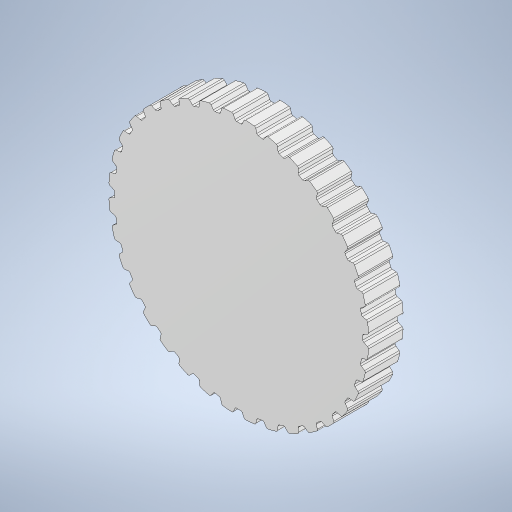
# Autodesk Inventor part: XL Pulley Generator
Saved by Autodesk Inventor 2023.4 (Build 274418000, 418)
## iProperties
RuleStatus: InUse
Created: 2022-06-22
Part Number: XL Pulley Generator
Material: UHMW, White
Document SubType Name: Modeling
Designer: Nathan Cai
Density: 0.94 g/cm^3
Appearance: Smooth - White
Mass: 3.49489 g
Surface Area: 67.8029 cm^2
Volume: 3.75794 cm^3
Author: Nathan Cai
Autodesk Inventor part; units mm, degrees
ref_plane "YZ Plane" through (0, 0, 0) normal (1, 0, 0) x (0, 1, 0)
ref_plane "XZ Plane" through (0, 0, 0) normal (0, 1, 0) x (-1, 0, 0)
ref_plane "XY Plane" through (0, 0, 0) normal (0, 0, 1) x (1, 0, 0)
sketch "Sketch2" plane through (0, 0, 0) normal (0, 0, 1) x (1, 0, 0)
  circle A0 centre (0, 0) radius 29.1063 construction
  circle A1 centre (0, 0) radius 28.5913
  dimension "Pd" = 58.2125
  dimension "OD" = 57.1825
  constraints: 2 centre point, 2 coincident
  measures "Pd" diameter of A0
  measures "OD" diameter of A1
extrude "Extrusion3" add sketch "Sketch2" along normal blind 7.62
sketch "Sketch3" plane through (0, 0, 7.62) normal (0, 0, 1) x (1, 0, 0)
  line L0 (0, 0) -> (0, 28.5913) construction
  circle A0 centre (0, 0) radius 28.5913 projected
  line L1 (0, 0) -> (4.9648, 28.1569) construction
  circle A1 centre (0, 0) radius 27.3213
  line L2 (0.8063, 27.5368) -> (1.1766, 28.3308)
  line L3 (1.2846, 28.5624) -> (0, 0) construction
  arc A2 (1.5415, 28.5497) -> (1.1766, 28.3308) centre (1.521, 28.1702) ccw
  arc A3 (0.4556, 27.3175) -> (0.8063, 27.5368) centre (0.4619, 27.6974) ccw
  circle A4 centre (0, 0) radius 28.5913 projected
  line L4 (-0.8063, 27.5368) -> (-1.1766, 28.3308)
  arc A5 (-1.1766, 28.3308) -> (-1.5415, 28.5497) centre (-1.521, 28.1702) ccw
  arc A6 (-0.8063, 27.5368) -> (-0.4556, 27.3175) centre (-0.4619, 27.6974) ccw
  point P0 (2.6792, 27.1896)
  point P1 (1.5415, 28.5497)
  point P2 (-1.5415, 28.5497)
  point P3 (-0.4556, 27.3175)
  dimension "d29" = 10
  dimension "d30" = 54.6425
  dimension "d31" = 25
  dimension "d33" = 2.575
  dimension "d34" = 0.76
  dimension "d35" = 0.76
  constraints: 14 point on circle, 10 end point, 6 symmetric about line, 5 centre point, 4 tangent, 1 coincident, 1 point on line, 1 vertical, 2 other
  measures "d29" angle of L0 L1
  measures "d30" diameter of A1
  measures "d31" angle of L0 L2
  measures "d33" angle of L0 L3
  measures "d34" diameter of A2
  measures "d35" diameter of A3
extrude "Extrusion4" cut sketch "Sketch3" against normal through all contours A2 L2 A3 A1 A6 L4 A5 A0 picked at (0.0506, 28.1647)
pattern_circular "Circular Pattern2" count 36 over 360 about axis through (0, 0, 0) along (0, 0, 1) of "Extrusion4"
equation "\"pitch\" = 5.08"
equation "\"width\" = 7.62"
equation "\"T_angle\" = 50deg"
equation "\"T_ht\" = 1.27"
equation "\"r1\" = 0.38"
equation "\"r2\" = 0.38"
equation "\"T_hs\" = 2.3"
equation "\"T_s\" = 2.57"
body "Solid3"
